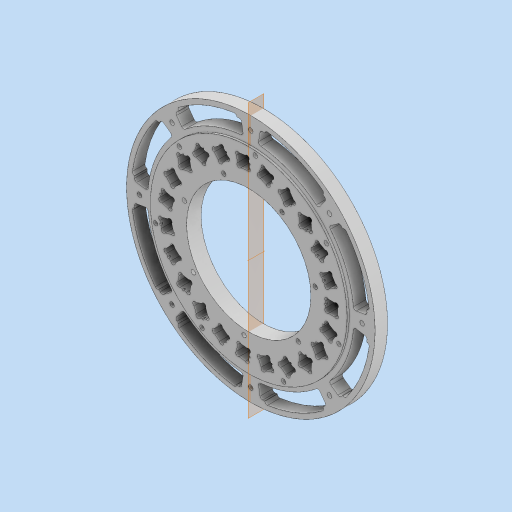
# Autodesk Inventor part: Ring_1050
Saved by Autodesk Inventor 2024.2 (Build 282272000, 272)
## iProperties
Created: 2025-04-23
Part Number: Ring_1050
Material: Generic
Document SubType Name: Modeling
Designer: 23661194
Density: 1 g/cm^3
Appearance: Default
Author: 23661194
Autodesk Inventor part; units mm, degrees
ref_plane "XZ Plane" through (0, 0, 0) normal (0, 1, 0) x (-1, 0, 0)
ref_plane "XY Plane" through (0, 0, 0) normal (0, 0, 1) x (1, 0, 0)
sketch "Shim Tray Slot_1" plane through (0, 0, 0) normal (0, 0, 1) x (1, 0, 0)
  line L0 (30.092, 109.0254) -> (29.9458, 108.3375)
  line L1 (33.5758, 105.3229) -> (31.6829, 97.1237)
  line L2 (-33.5758, 105.3229) -> (-31.6821, 97.1202)
  line L3 (-30.092, 109.0254) -> (-29.9458, 108.3375)
  arc A0 (-32.2001, 107.689) -> (-33.5758, 105.3229) centre (-31.6271, 105.7728) ccw
  arc A1 (29.147, 95.658) -> (-29.1504, 95.657) centre (0, 0) ccw
  arc A2 (28.6337, 111.3782) -> (-28.6337, 111.3782) centre (0, 0) ccw
  arc A3 (-29.9458, 108.3375) -> (-32.2001, 107.689) centre (0, 0) ccw
  arc A4 (32.2001, 107.689) -> (29.9458, 108.3375) centre (0, 0) ccw
  arc A5 (-28.6337, 111.3782) -> (-30.092, 109.0254) centre (-28.1357, 109.4412) ccw
  arc A6 (-31.6821, 97.1202) -> (-29.1504, 95.657) centre (-29.7334, 97.5701) ccw
  arc A7 (29.147, 95.658) -> (31.6829, 97.1237) centre (29.7309, 97.5743) ccw
  arc A8 (33.5758, 105.3229) -> (32.2001, 107.689) centre (31.6271, 105.7728) ccw
  arc A9 (30.092, 109.0254) -> (28.6337, 111.3782) centre (28.1357, 109.4412) ccw
  line L4 (0, 0) -> (0, 107.5)
  arc A10 (33.9656, 105.2329) -> (32.3146, 108.0722) centre (31.6271, 105.7728) ccw
  line L5 (33.9656, 105.2329) -> (32.0726, 97.0337)
  arc A11 (29.0304, 95.2754) -> (32.0726, 97.0337) centre (29.7309, 97.5743) ccw
  arc A12 (29.0304, 95.2754) -> (-29.0338, 95.2743) centre (0, 0) ccw
  arc A13 (-32.0718, 97.0302) -> (-29.0338, 95.2743) centre (-29.7334, 97.5701) ccw
  line L6 (-32.0718, 97.0302) -> (-33.9656, 105.2329)
  arc A14 (-32.3146, 108.0722) -> (-33.9656, 105.2329) centre (-31.6271, 105.7728) ccw
  arc A15 (-30.4152, 108.6221) -> (-32.3146, 108.0722) centre (0, 0) ccw
  line L7 (-30.4152, 108.6221) -> (-30.4833, 108.9422)
  arc A16 (-28.7333, 111.7656) -> (-30.4833, 108.9422) centre (-28.1357, 109.4412) ccw
  arc A17 (28.7333, 111.7656) -> (-28.7333, 111.7656) centre (0, 0) ccw
  arc A18 (30.4833, 108.9422) -> (28.7333, 111.7656) centre (28.1357, 109.4412) ccw
  line L8 (30.4833, 108.9422) -> (30.4152, 108.6221)
  arc A19 (32.3146, 108.0722) -> (30.4152, 108.6221) centre (0, 0) ccw
  dimension "d150" = 22.5
  dimension "d159" = 0.4
  measures "d159" radial gap between concentric circles of A2 A17
sketch "Sketch1" plane through (0, 0, 0) normal (0, 0, 1) x (1, 0, 0)
  circle A0 centre (0, 0) radius 60
  circle A1 centre (0, 0) radius 120
  circle A2 centre (0, 0) radius 95
  dimension "d0" = 120
  dimension "d1" = 240
  dimension "d2" = 190
  constraints: 5 coincident, 3 centre point
  measures "d0" diameter of A0
  measures "d1" diameter of A1
  measures "d2" diameter of A2
extrude "Extrusion1" add sketch "Sketch1" along normal blind 12 contours A1 | A2
extrude "Extrusion2" add sketch "Sketch1" along normal blind 14 contours A2
sketch "Sketch2" plane through (0, 0, 14) normal (0, 0, 1) x (1, 0, 0)
  circle A0 centre (0, 0) radius 80.0067
  circle A1 centre (0, 0) radius 60 projected
  line L0 (80.0067, 0) -> (0, 0)
  line L1 (77.0399, 21.5856) -> (0, 0)
  line L2 (68.3593, 41.5702) -> (0, 0)
  line L3 (54.6089, 58.4718) -> (0, 0)
  line L4 (36.8083, 71.0368) -> (0, 0)
  line L5 (16.2779, 78.3333) -> (0, 0)
  line L6 (-5.4599, 79.8202) -> (0, 0)
  line L7 (-26.7926, 75.3872) -> (0, 0)
  line L8 (-46.1383, 65.3631) -> (0, 0)
  line L9 (-62.0621, 50.4913) -> (0, 0)
  line L10 (-73.3831, 31.8748) -> (0, 0)
  line L11 (-79.2616, 10.8942) -> (0, 0)
  line L12 (-79.2616, -10.8942) -> (0, 0)
  line L13 (-73.3831, -31.8748) -> (0, 0)
  line L14 (-62.0621, -50.4913) -> (0, 0)
  line L15 (-46.1383, -65.3631) -> (0, 0)
  line L16 (-26.7926, -75.3872) -> (0, 0)
  line L17 (-5.4599, -79.8202) -> (0, 0)
  line L18 (16.2779, -78.3333) -> (0, 0)
  line L19 (36.8083, -71.0368) -> (0, 0)
  line L20 (54.6089, -58.4718) -> (0, 0)
  line L21 (68.3593, -41.5702) -> (0, 0)
  line L22 (77.0399, -21.5856) -> (0, 0)
  line L23 (-168, 0) -> (168, 0) projected
  line L24 (85.9467, 5.94) -> (74.0667, 5.94)
  line L25 (74.0667, 5.94) -> (74.0667, -5.94)
  line L26 (74.0667, -5.94) -> (85.9467, -5.94)
  line L27 (85.9467, -5.94) -> (85.9467, 5.94)
  line L28 (85.9467, 5.94) -> (74.0667, -5.94) construction
  line L29 (74.0667, 5.94) -> (85.9467, -5.94) construction
  circle A2 centre (80.0067, 0) radius 2
  circle A3 centre (75.4797, -4.527) radius 2.1
  circle A4 centre (84.5337, -4.527) radius 2.1
  circle A5 centre (84.5337, 4.527) radius 2.1
  circle A6 centre (75.4797, 4.527) radius 2.1
  circle A7 centre (73.7067, 0) radius 0.75
  line L30 (73.7067, 0) -> (80.0067, 0)
  line L31 (79.0288, 29.7471) -> (68.8783, 23.5745)
  line L32 (68.8783, 23.5745) -> (75.0509, 13.424)
  line L33 (75.0509, 13.424) -> (85.2015, 19.5966)
  line L34 (85.2015, 19.5966) -> (79.0288, 29.7471)
  line L35 (79.0288, 29.7471) -> (75.0509, 13.424) construction
  line L36 (68.8783, 23.5745) -> (85.2015, 19.5966) construction
  circle A8 centre (77.0399, 21.5856) radius 2
  circle A9 centre (75.5241, 15.3654) radius 2.1
  circle A10 centre (83.26, 20.0698) radius 2.1
  circle A11 centre (78.5557, 27.8057) radius 2.1
  circle A12 centre (70.8198, 23.1014) radius 2.1
  circle A13 centre (71.657, 18.3122) radius 0.75
  line L37 (71.657, 18.3122) -> (77.0399, 21.5856)
  line L38 (65.8181, 49.577) -> (60.3525, 39.029)
  line L39 (60.3525, 39.029) -> (70.9006, 33.5634)
  line L40 (70.9006, 33.5634) -> (76.3661, 44.1115)
  line L41 (76.3661, 44.1115) -> (65.8181, 49.577)
  line L42 (65.8181, 49.577) -> (70.9006, 33.5634) construction
  line L43 (60.3525, 39.029) -> (76.3661, 44.1115) construction
  circle A14 centre (68.3593, 41.5702) radius 2
  circle A15 centre (70.2961, 35.468) radius 2.1
  circle A16 centre (74.4615, 43.507) radius 2.1
  circle A17 centre (66.4226, 47.6724) radius 2.1
  circle A18 centre (62.2571, 39.6335) radius 2.1
  circle A19 centre (65.4609, 35.9765) radius 0.75
  line L44 (65.4609, 35.9765) -> (68.3593, 41.5702)
  line L45 (48.2773, 63.9926) -> (49.0881, 52.1403)
  line L46 (49.0881, 52.1403) -> (60.9404, 52.951)
  line L47 (60.9404, 52.951) -> (60.1296, 64.8033)
  line L48 (60.1296, 64.8033) -> (48.2773, 63.9926)
  line L49 (48.2773, 63.9926) -> (60.9404, 52.951) construction
  line L50 (49.0881, 52.1403) -> (60.1296, 64.8033) construction
  circle A20 centre (54.6089, 58.4718) radius 2
  circle A21 centre (59.4342, 54.2643) radius 2.1
  circle A22 centre (58.8164, 63.2972) radius 2.1
  circle A23 centre (49.7835, 62.6793) radius 2.1
  circle A24 centre (50.4013, 53.6464) radius 2.1
  circle A25 centre (55.0388, 52.1865) radius 0.75
  line L51 (55.0388, 52.1865) -> (54.6089, 58.4718)
  line L52 (28.53, 72.4641) -> (35.381, 62.7585)
  line L53 (35.381, 62.7585) -> (45.0866, 69.6095)
  line L54 (45.0866, 69.6095) -> (38.2356, 79.3151)
  line L55 (38.2356, 79.3151) -> (28.53, 72.4641)
  line L56 (28.53, 72.4641) -> (45.0866, 69.6095) construction
  line L57 (35.381, 62.7585) -> (38.2356, 79.3151) construction
  circle A26 centre (36.8083, 71.0368) radius 2
  circle A27 centre (43.1174, 69.949) radius 2.1
  circle A28 centre (37.8961, 77.3459) radius 2.1
  circle A29 centre (30.4992, 72.1246) radius 2.1
  circle A30 centre (35.7205, 64.7277) radius 2.1
  circle A31 centre (40.4414, 65.8899) radius 0.75
  line L58 (40.4414, 65.8899) -> (36.8083, 71.0368)
  line L59 (8.4631, 75.2516) -> (19.3596, 70.5186)
  line L60 (19.3596, 70.5186) -> (24.0926, 81.4151)
  line L61 (24.0926, 81.4151) -> (13.1961, 86.1481)
  line L62 (13.1961, 86.1481) -> (8.4631, 75.2516)
  line L63 (8.4631, 75.2516) -> (24.0926, 81.4151) construction
  line L64 (19.3596, 70.5186) -> (13.1961, 86.1481) construction
  circle A32 centre (16.2779, 78.3333) radius 2
  circle A33 centre (22.2336, 80.682) radius 2.1
  circle A34 centre (13.9292, 84.2891) radius 2.1
  circle A35 centre (10.3221, 75.9847) radius 2.1
  circle A36 centre (18.6265, 72.3775) radius 2.1
  circle A37 centre (22.0563, 75.8234) radius 0.75
  line L65 (22.0563, 75.8234) -> (16.2779, 78.3333)
  line L66 (-10.5357, 73.1267) -> (1.2337, 74.7444)
  line L67 (1.2337, 74.7444) -> (-0.384, 86.5137)
  line L68 (-0.384, 86.5137) -> (-12.1534, 84.8961)
  line L69 (-12.1534, 84.8961) -> (-10.5357, 73.1267)
  line L70 (-10.5357, 73.1267) -> (-0.384, 86.5137) construction
  line L71 (1.2337, 74.7444) -> (-12.1534, 84.8961) construction
  circle A38 centre (-5.4599, 79.8202) radius 2
  circle A39 centre (-1.5914, 84.9215) radius 2.1
  circle A40 centre (-10.5611, 83.6886) radius 2.1
  circle A41 centre (-9.3283, 74.719) radius 2.1
  circle A42 centre (-0.3586, 75.9518) radius 2.1
  circle A43 centre (0.7815, 80.6781) radius 0.75
  line L72 (0.7815, 80.6781) -> (-5.4599, 79.8202)
  line L73 (-27.6517, 67.0308) -> (-18.4362, 74.5282)
  line L74 (-18.4362, 74.5282) -> (-25.9336, 83.7436)
  line L75 (-25.9336, 83.7436) -> (-35.149, 76.2463)
  line L76 (-35.149, 76.2463) -> (-27.6517, 67.0308)
  line L77 (-27.6517, 67.0308) -> (-25.9336, 83.7436) construction
  line L78 (-18.4362, 74.5282) -> (-35.149, 76.2463) construction
  circle A44 centre (-26.7926, 75.3872) radius 2
  circle A45 centre (-26.1379, 81.7558) radius 2.1
  circle A46 centre (-33.1612, 76.0419) radius 2.1
  circle A47 centre (-27.4473, 69.0186) radius 2.1
  circle A48 centre (-20.424, 74.7325) radius 2.1
  circle A49 centre (-21.9056, 79.3631) radius 0.75
  line L79 (-21.9056, 79.3631) -> (-26.7926, 75.3872)
  line L80 (-42.5305, 57.7769) -> (-38.5521, 68.9709)
  line L81 (-38.5521, 68.9709) -> (-49.7462, 72.9493)
  line L82 (-49.7462, 72.9493) -> (-53.7245, 61.7553)
  line L83 (-53.7245, 61.7553) -> (-42.5305, 57.7769)
  line L84 (-42.5305, 57.7769) -> (-49.7462, 72.9493) construction
  line L85 (-38.5521, 68.9709) -> (-53.7245, 61.7553) construction
  circle A50 centre (-46.1383, 65.3631) radius 2
  circle A51 centre (-48.8879, 71.1447) radius 2.1
  circle A52 centre (-51.9199, 62.6135) radius 2.1
  circle A53 centre (-43.3887, 59.5815) radius 2.1
  circle A54 centre (-40.3567, 68.1127) radius 2.1
  circle A55 centre (-44.0286, 71.2993) radius 0.75
  line L86 (-44.0286, 71.2993) -> (-46.1383, 65.3631)
  line L87 (-55.0378, 45.8841) -> (-57.4549, 57.5156)
  line L88 (-57.4549, 57.5156) -> (-69.0864, 55.0985)
  line L89 (-69.0864, 55.0985) -> (-66.6694, 43.467)
  line L90 (-66.6694, 43.467) -> (-55.0378, 45.8841)
  line L91 (-55.0378, 45.8841) -> (-69.0864, 55.0985) construction
  line L92 (-57.4549, 57.5156) -> (-66.6694, 43.467) construction
  circle A56 centre (-62.0621, 50.4913) radius 2
  circle A57 centre (-67.4155, 54.0026) radius 2.1
  circle A58 centre (-65.5734, 45.1379) radius 2.1
  circle A59 centre (-56.7088, 46.98) radius 2.1
  circle A60 centre (-58.5509, 55.8446) radius 2.1
  circle A61 centre (-63.3439, 56.6595) radius 0.75
  line L93 (-63.3439, 56.6595) -> (-62.0621, 50.4913)
  line L94 (-64.9876, 31.588) -> (-73.0963, 40.2703)
  line L95 (-73.0963, 40.2703) -> (-81.7786, 32.1616)
  line L96 (-81.7786, 32.1616) -> (-73.6699, 23.4792)
  line L97 (-73.6699, 23.4792) -> (-64.9876, 31.588)
  line L98 (-64.9876, 31.588) -> (-81.7786, 32.1616) construction
  line L99 (-73.0963, 40.2703) -> (-73.6699, 23.4792) construction
  circle A62 centre (-73.3831, 31.8748) radius 2
  circle A63 centre (-79.7815, 32.0933) radius 2.1
  circle A64 centre (-73.6017, 25.4764) radius 2.1
  circle A65 centre (-66.9847, 31.6562) radius 2.1
  circle A66 centre (-73.1645, 38.2732) radius 2.1
  circle A67 centre (-77.6832, 36.479) radius 0.75
  line L100 (-77.6832, 36.479) -> (-73.3831, 31.8748)
  line L101 (-71.9392, 15.0114) -> (-83.3787, 18.2166)
  line L102 (-83.3787, 18.2166) -> (-86.5839, 6.7771)
  line L103 (-86.5839, 6.7771) -> (-75.1444, 3.5719)
  line L104 (-75.1444, 3.5719) -> (-71.9392, 15.0114)
  line L105 (-71.9392, 15.0114) -> (-86.5839, 6.7771) construction
  line L106 (-83.3787, 18.2166) -> (-75.1444, 3.5719) construction
  circle A68 centre (-79.2616, 10.8942) radius 2
  circle A69 centre (-84.842, 7.7565) radius 2.1
  circle A70 centre (-76.1238, 5.3138) radius 2.1
  circle A71 centre (-73.6811, 14.032) radius 2.1
  circle A72 centre (-82.3993, 16.4747) radius 2.1
  circle A73 centre (-85.3279, 12.594) radius 0.75
  line L107 (-85.3279, 12.594) -> (-79.2616, 10.8942)
  line L108 (-75.1444, -3.5719) -> (-86.5839, -6.7771)
  line L109 (-86.5839, -6.7771) -> (-83.3787, -18.2166)
  line L110 (-83.3787, -18.2166) -> (-71.9392, -15.0114)
  line L111 (-71.9392, -15.0114) -> (-75.1444, -3.5719)
  line L112 (-75.1444, -3.5719) -> (-83.3787, -18.2166) construction
  line L113 (-86.5839, -6.7771) -> (-71.9392, -15.0114) construction
  circle A74 centre (-79.2616, -10.8942) radius 2
  circle A75 centre (-82.3993, -16.4747) radius 2.1
  circle A76 centre (-73.6811, -14.032) radius 2.1
  circle A77 centre (-76.1238, -5.3138) radius 2.1
  circle A78 centre (-84.842, -7.7565) radius 2.1
  circle A79 centre (-85.3279, -12.594) radius 0.75
  line L114 (-85.3279, -12.594) -> (-79.2616, -10.8942)
  line L115 (-73.6699, -23.4792) -> (-81.7786, -32.1616)
  line L116 (-81.7786, -32.1616) -> (-73.0963, -40.2703)
  line L117 (-73.0963, -40.2703) -> (-64.9876, -31.588)
  line L118 (-64.9876, -31.588) -> (-73.6699, -23.4792)
  line L119 (-73.6699, -23.4792) -> (-73.0963, -40.2703) construction
  line L120 (-81.7786, -32.1616) -> (-64.9876, -31.588) construction
  circle A80 centre (-73.3831, -31.8748) radius 2
  circle A81 centre (-73.1645, -38.2732) radius 2.1
  circle A82 centre (-66.9847, -31.6562) radius 2.1
  circle A83 centre (-73.6017, -25.4764) radius 2.1
  circle A84 centre (-79.7815, -32.0934) radius 2.1
  circle A85 centre (-77.6832, -36.479) radius 0.75
  line L121 (-77.6832, -36.479) -> (-73.3831, -31.8748)
  line L122 (-66.6694, -43.467) -> (-69.0864, -55.0985)
  line L123 (-69.0864, -55.0985) -> (-57.4549, -57.5156)
  line L124 (-57.4549, -57.5156) -> (-55.0378, -45.8841)
  line L125 (-55.0378, -45.8841) -> (-66.6694, -43.467)
  line L126 (-66.6694, -43.467) -> (-57.4549, -57.5156) construction
  line L127 (-69.0864, -55.0985) -> (-55.0378, -45.8841) construction
  circle A86 centre (-62.0621, -50.4913) radius 2
  circle A87 centre (-58.5509, -55.8446) radius 2.1
  circle A88 centre (-56.7088, -46.98) radius 2.1
  circle A89 centre (-65.5734, -45.1379) radius 2.1
  circle A90 centre (-67.4155, -54.0026) radius 2.1
  circle A91 centre (-63.3439, -56.6595) radius 0.75
  line L128 (-63.3439, -56.6595) -> (-62.0621, -50.4913)
  line L129 (-53.7245, -61.7553) -> (-49.7462, -72.9493)
  line L130 (-49.7462, -72.9493) -> (-38.5521, -68.9709)
  line L131 (-38.5521, -68.9709) -> (-42.5305, -57.7769)
  line L132 (-42.5305, -57.7769) -> (-53.7245, -61.7553)
  line L133 (-53.7245, -61.7553) -> (-38.5521, -68.9709) construction
  line L134 (-49.7462, -72.9493) -> (-42.5305, -57.7769) construction
  circle A92 centre (-46.1383, -65.3631) radius 2
  circle A93 centre (-40.3567, -68.1127) radius 2.1
  circle A94 centre (-43.3887, -59.5815) radius 2.1
  circle A95 centre (-51.9199, -62.6135) radius 2.1
  circle A96 centre (-48.8879, -71.1447) radius 2.1
  circle A97 centre (-44.0286, -71.2993) radius 0.75
  line L135 (-44.0286, -71.2993) -> (-46.1383, -65.3631)
  line L136 (-35.149, -76.2463) -> (-25.9336, -83.7436)
  line L137 (-25.9336, -83.7436) -> (-18.4362, -74.5282)
  line L138 (-18.4362, -74.5282) -> (-27.6517, -67.0308)
  line L139 (-27.6517, -67.0308) -> (-35.149, -76.2463)
  line L140 (-35.149, -76.2463) -> (-18.4362, -74.5282) construction
  line L141 (-25.9336, -83.7436) -> (-27.6517, -67.0308) construction
  circle A98 centre (-26.7926, -75.3872) radius 2
  circle A99 centre (-20.424, -74.7325) radius 2.1
  circle A100 centre (-27.4473, -69.0186) radius 2.1
  circle A101 centre (-33.1612, -76.0419) radius 2.1
  circle A102 centre (-26.1379, -81.7558) radius 2.1
  circle A103 centre (-21.9056, -79.3631) radius 0.75
  line L142 (-21.9056, -79.3631) -> (-26.7926, -75.3872)
  line L143 (-12.1534, -84.8961) -> (-0.384, -86.5137)
  line L144 (-0.384, -86.5137) -> (1.2337, -74.7444)
  line L145 (1.2337, -74.7444) -> (-10.5357, -73.1267)
  line L146 (-10.5357, -73.1267) -> (-12.1534, -84.8961)
  line L147 (-12.1534, -84.8961) -> (1.2337, -74.7444) construction
  line L148 (-0.384, -86.5137) -> (-10.5357, -73.1267) construction
  circle A104 centre (-5.4599, -79.8202) radius 2
  circle A105 centre (-0.3586, -75.9518) radius 2.1
  circle A106 centre (-9.3283, -74.719) radius 2.1
  circle A107 centre (-10.5611, -83.6886) radius 2.1
  circle A108 centre (-1.5914, -84.9215) radius 2.1
  circle A109 centre (0.7815, -80.6781) radius 0.75
  line L149 (0.7815, -80.6781) -> (-5.4599, -79.8202)
  line L150 (13.1961, -86.1481) -> (24.0926, -81.4151)
  line L151 (24.0926, -81.4151) -> (19.3596, -70.5186)
  line L152 (19.3596, -70.5186) -> (8.4631, -75.2516)
  line L153 (8.4631, -75.2516) -> (13.1961, -86.1481)
  line L154 (13.1961, -86.1481) -> (19.3596, -70.5186) construction
  line L155 (24.0926, -81.4151) -> (8.4631, -75.2516) construction
  circle A110 centre (16.2779, -78.3333) radius 2
  circle A111 centre (18.6265, -72.3775) radius 2.1
  circle A112 centre (10.3221, -75.9847) radius 2.1
  circle A113 centre (13.9292, -84.2891) radius 2.1
  circle A114 centre (22.2336, -80.682) radius 2.1
  circle A115 centre (22.0563, -75.8234) radius 0.75
  line L156 (22.0563, -75.8234) -> (16.2779, -78.3333)
  line L157 (38.2356, -79.3151) -> (45.0866, -69.6095)
  line L158 (45.0866, -69.6095) -> (35.381, -62.7585)
  line L159 (35.381, -62.7585) -> (28.53, -72.4641)
  line L160 (28.53, -72.4641) -> (38.2356, -79.3151)
  line L161 (38.2356, -79.3151) -> (35.381, -62.7585) construction
  line L162 (45.0866, -69.6095) -> (28.53, -72.4641) construction
  circle A116 centre (36.8083, -71.0368) radius 2
  circle A117 centre (35.7205, -64.7277) radius 2.1
  circle A118 centre (30.4992, -72.1246) radius 2.1
  circle A119 centre (37.8961, -77.3459) radius 2.1
  circle A120 centre (43.1174, -69.949) radius 2.1
  circle A121 centre (40.4414, -65.8899) radius 0.75
  line L163 (40.4414, -65.8899) -> (36.8083, -71.0368)
  line L164 (60.1296, -64.8033) -> (60.9404, -52.951)
  line L165 (60.9404, -52.951) -> (49.0881, -52.1403)
  line L166 (49.0881, -52.1403) -> (48.2773, -63.9926)
  line L167 (48.2773, -63.9926) -> (60.1296, -64.8033)
  line L168 (60.1296, -64.8033) -> (49.0881, -52.1403) construction
  line L169 (60.9404, -52.951) -> (48.2773, -63.9926) construction
  circle A122 centre (54.6089, -58.4718) radius 2
  circle A123 centre (50.4013, -53.6464) radius 2.1
  circle A124 centre (49.7835, -62.6793) radius 2.1
  circle A125 centre (58.8164, -63.2972) radius 2.1
  circle A126 centre (59.4342, -54.2643) radius 2.1
  circle A127 centre (55.0388, -52.1865) radius 0.75
  line L170 (55.0388, -52.1865) -> (54.6089, -58.4718)
  line L171 (76.3661, -44.1115) -> (70.9006, -33.5634)
  line L172 (70.9006, -33.5634) -> (60.3525, -39.029)
  line L173 (60.3525, -39.029) -> (65.8181, -49.577)
  line L174 (65.8181, -49.577) -> (76.3661, -44.1115)
  line L175 (76.3661, -44.1115) -> (60.3525, -39.029) construction
  line L176 (70.9006, -33.5634) -> (65.8181, -49.577) construction
  circle A128 centre (68.3593, -41.5702) radius 2
  circle A129 centre (62.2571, -39.6335) radius 2.1
  circle A130 centre (66.4226, -47.6724) radius 2.1
  circle A131 centre (74.4615, -43.507) radius 2.1
  circle A132 centre (70.2961, -35.468) radius 2.1
  circle A133 centre (65.4609, -35.9765) radius 0.75
  line L177 (65.4609, -35.9765) -> (68.3593, -41.5702)
  line L178 (85.2015, -19.5966) -> (75.0509, -13.424)
  line L179 (75.0509, -13.424) -> (68.8783, -23.5745)
  line L180 (68.8783, -23.5745) -> (79.0288, -29.7471)
  line L181 (79.0288, -29.7471) -> (85.2015, -19.5966)
  line L182 (85.2015, -19.5966) -> (68.8783, -23.5745) construction
  line L183 (75.0509, -13.424) -> (79.0288, -29.7471) construction
  circle A134 centre (77.0399, -21.5856) radius 2
  circle A135 centre (70.8198, -23.1014) radius 2.1
  circle A136 centre (78.5557, -27.8057) radius 2.1
  circle A137 centre (83.26, -20.0698) radius 2.1
  circle A138 centre (75.5241, -15.3654) radius 2.1
  circle A139 centre (71.657, -18.3122) radius 0.75
  line L184 (71.657, -18.3122) -> (77.0399, -21.5856)
  point P0 (76.4941, -28.2058)
  point P1 (80.5702, -27.2125)
  point P2 (83.6601, -22.1313)
  point P3 (82.6668, -18.0553)
  point P4 (77.5856, -14.9653)
  point P5 (73.5096, -15.9586)
  point P6 (70.4196, -21.0398)
  point P7 (71.4129, -25.1158)
  point P8 (61.7173, -41.6629)
  point P9 (64.4533, -46.9431)
  point P10 (68.452, -48.2122)
  point P11 (73.7322, -45.4763)
  point P12 (75.0013, -41.4775)
  point P13 (72.2654, -36.1973)
  point P14 (68.2666, -34.9282)
  point P15 (62.9864, -37.6642)
  point P16 (60.7379, -55.9106)
  point P17 (57.9808, -52.7486)
  point P18 (52.0477, -52.3427)
  point P19 (48.8856, -55.0999)
  point P20 (48.4798, -61.033)
  point P21 (51.2369, -64.195)
  point P22 (57.17, -64.6009)
  point P23 (60.3321, -61.8437)
  point P24 (30.2408, -70.0406)
  point P25 (30.9536, -74.1749)
  point P26 (35.8121, -77.6043)
  point P27 (39.9464, -76.8915)
  point P28 (43.3759, -72.033)
  point P29 (42.663, -67.8987)
  point P30 (37.8045, -64.4693)
  point P31 (33.6702, -65.1821)
  point P32 (12.0143, -83.4271)
  point P33 (15.917, -84.9662)
  point P34 (21.3717, -82.5969)
  point P35 (22.9107, -78.6941)
  point P36 (20.5415, -73.2395)
  point P37 (16.6387, -71.7005)
  point P38 (11.184, -74.0697)
  point P39 (9.645, -77.9725)
  point P40 (0.8297, -77.6833)
  point P41 (-1.7052, -74.3404)
  point P42 (-7.5968, -73.5307)
  point P43 (-10.9396, -76.0656)
  point P44 (-11.7494, -81.9572)
  point P45 (-9.2145, -85.3)
  point P46 (-3.3229, -86.1098)
  point P47 (0.0199, -83.5748)
  point P48 (-25.3505, -68.903)
  point P49 (-29.5238, -69.332)
  point P50 (-33.2769, -73.9451)
  point P51 (-32.8478, -78.1184)
  point P52 (-28.2347, -81.8715)
  point P53 (-24.0614, -81.4424)
  point P54 (-20.3084, -76.8293)
  point P55 (-20.7374, -72.656)
  point P56 (-52.7311, -64.5505)
  point P57 (-50.7396, -70.1541)
  point P58 (-46.9509, -71.9559)
  point P59 (-41.3473, -69.9644)
  point P60 (-39.5455, -66.1757)
  point P61 (-41.537, -60.5721)
  point P62 (-45.3257, -58.7703)
  point P63 (-50.9293, -60.7618)
  point P64 (-56.8513, -54.6111)
  point P65 (-55.6414, -48.7885)
  point P66 (-57.9423, -45.2805)
  point P67 (-63.7649, -44.0706)
  point P68 (-67.2729, -46.3715)
  point P69 (-68.4829, -52.194)
  point P70 (-66.1819, -55.7021)
  point P71 (-60.3594, -56.912)
  point P72 (-71.5019, -25.504)
  point P73 (-75.6947, -25.6473)
  point P74 (-79.7538, -29.9935)
  point P75 (-79.6106, -34.1864)
  point P76 (-75.2643, -38.2455)
  point P77 (-71.0715, -38.1023)
  point P78 (-67.0124, -33.756)
  point P79 (-67.1556, -29.5631)
  point P80 (-74.3441, -6.4284)
  point P81 (-78.0009, -4.3723)
  point P82 (-83.7274, -5.9768)
  point P83 (-85.7835, -9.6336)
  point P84 (-84.179, -15.3601)
  point P85 (-80.5222, -17.4162)
  point P86 (-74.7957, -15.8117)
  point P87 (-72.7396, -12.1549)
  point P88 (-72.7396, 12.1549)
  point P89 (-74.7957, 15.8117)
  point P90 (-80.5222, 17.4162)
  point P91 (-84.179, 15.3601)
  point P92 (-85.7835, 9.6336)
  point P93 (-83.7274, 5.9768)
  point P94 (-78.0009, 4.3723)
  point P95 (-74.3441, 6.4284)
  point P96 (-67.1556, 29.5632)
  point P97 (-67.0124, 33.756)
  point P98 (-71.0715, 38.1023)
  point P99 (-75.2643, 38.2455)
  point P100 (-79.6106, 34.1864)
  point P101 (-79.7538, 29.9935)
  point P102 (-75.6947, 25.6473)
  point P103 (-71.5018, 25.504)
  point P104 (-57.9423, 45.2805)
  point P105 (-55.6414, 48.7885)
  point P106 (-56.8513, 54.6111)
  point P107 (-60.3594, 56.912)
  point P108 (-66.1819, 55.7021)
  point P109 (-68.4829, 52.194)
  point P110 (-67.2729, 46.3715)
  point P111 (-63.7649, 44.0706)
  point P112 (-45.3257, 58.7703)
  point P113 (-41.537, 60.5721)
  point P114 (-39.5455, 66.1757)
  point P115 (-41.3473, 69.9644)
  point P116 (-46.9509, 71.9559)
  point P117 (-50.7396, 70.1541)
  point P118 (-52.7311, 64.5505)
  point P119 (-50.9293, 60.7618)
  point P120 (-20.7374, 72.656)
  point P121 (-20.3084, 76.8293)
  point P122 (-24.0614, 81.4424)
  point P123 (-28.2347, 81.8715)
  point P124 (-32.8478, 78.1184)
  point P125 (-33.2769, 73.9451)
  point P126 (-29.5238, 69.332)
  point P127 (-25.3505, 68.903)
  point P128 (-10.9396, 76.0656)
  point P129 (-7.5968, 73.5307)
  point P130 (-1.7052, 74.3404)
  point P131 (0.8297, 77.6833)
  point P132 (0.0199, 83.5748)
  point P133 (-3.3229, 86.1098)
  point P134 (-9.2145, 85.3)
  point P135 (-11.7494, 81.9572)
  point P136 (9.645, 77.9725)
  point P137 (11.184, 74.0697)
  point P138 (16.6387, 71.7005)
  point P139 (20.5415, 73.2395)
  point P140 (22.9107, 78.6941)
  point P141 (21.3717, 82.5969)
  point P142 (15.917, 84.9662)
  point P143 (12.0143, 83.4271)
  point P144 (30.2408, 70.0406)
  point P145 (33.6702, 65.1821)
  point P146 (37.8045, 64.4693)
  point P147 (42.663, 67.8987)
  point P148 (43.3759, 72.033)
  point P149 (39.9464, 76.8915)
  point P150 (35.8121, 77.6043)
  point P151 (30.9536, 74.1749)
  point P152 (60.7379, 55.9106)
  point P153 (60.3321, 61.8437)
  point P154 (57.17, 64.6009)
  point P155 (51.2369, 64.195)
  point P156 (48.4798, 61.033)
  point P157 (48.8856, 55.0999)
  point P158 (52.0477, 52.3427)
  point P159 (57.9808, 52.7486)
  point P160 (72.2654, 36.1973)
  point P161 (75.0013, 41.4775)
  point P162 (73.7322, 45.4763)
  point P163 (68.452, 48.2122)
  point P164 (64.4533, 46.9431)
  point P165 (61.7173, 41.6629)
  point P166 (62.9864, 37.6642)
  point P167 (68.2666, 34.9282)
  point P168 (71.4129, 25.1158)
  point P169 (70.4196, 21.0398)
  point P170 (73.5096, 15.9586)
  point P171 (77.5856, 14.9653)
  point P172 (82.6668, 18.0553)
  point P173 (83.6601, 22.1313)
  point P174 (80.5702, 27.2125)
  point P175 (76.4941, 28.2058)
  point P176 (77.0333, 5.94)
  point P177 (74.0667, 2.9735)
  point P178 (74.0667, -2.9735)
  point P179 (77.0333, -5.94)
  point P180 (82.9802, -5.94)
  point P181 (85.9467, -2.9735)
  point P182 (85.9467, 2.9735)
  point P183 (82.9802, 5.94)
  dimension "d7" = 160.0135
  dimension "d93" = -31.304
  dimension "d94" = -62.609
  dimension "d95" = -93.913
  dimension "d96" = -125.217
  dimension "d97" = -156.522
  dimension "d98" = -187.826
  dimension "d99" = -219.13
  dimension "d100" = -250.435
  dimension "d101" = -281.739
  dimension "d103" = -344.348
  dimension "d104" = -15.652
  dimension "d105" = -46.957
  dimension "d106" = -78.261
  dimension "d107" = -109.565
  dimension "d108" = -140.87
  dimension "d109" = -172.174
  dimension "d110" = -203.478
  dimension "d111" = -234.783
  dimension "d112" = -266.087
  dimension "d113" = -297.391
  dimension "d114" = -328.696
  dimension "d10" = 360
  dimension "d92" = 0
  dimension "d102" = -313.043
  constraints: 46 end point, 1 coincident, 1 horizontal, 1 horizontal alignment, 96 other
  measures "d92" vertical extent of L0
extrude "Extrusion3" cut sketch "Sketch2" against normal blind 12 contours L0 A2 A0 | L23 A2 A0 | A0 A2 L0 | A0 A2 L23 | A2 L0 A7 L25 A6 L24 A0 | A0 L24 A5 L27 L23 A2 | A2 L23 L27 A4 L26 A0 | A0 L26 A3 L25 A7 L0 A2 | A7 L25 L0 | L0 L25 A7 | L33 A9 L32 A13 L37 A8 A0 | A0 A8 L31 A11 L34 A10 L33 | A5 L27 L24 | L24 L27 A5 | A6 L25 L24 | L24 L25 A6 | L178 A137 L181 A136 L180 A0 A134 | A0 A134 L184 A139 L179 A138 L178 | A3 L25 L26 | L26 L25 A3 | A4 L27 L26 | L26 L27 A4 | A8 L37 A0 | A0 A8 | A9 L32 L33 | L33 L32 A9 | A10 L34 L33 | L33 L34 A10 | A134 A0 | A0 L184 A134 | A137 L181 L178 | L178 L181 A137 | A138 L179 L178 | L178 L179 A138 | L1 A8 A0 | L37 A8 L1 | L37 A13 L32 L1 A8 | A0 A134 L22 | L22 A134 L184 | A134 L22 L179 A139 L184 | A8 L1 L32 A12 L31 A0 | L37 L32 A13 | A13 L32 L37 | A11 L31 L34 | L34 L31 A11 | A0 L180 A135 L179 L22 A134 | L184 L179 A139 | A139 L179 L184 | A136 L180 L181 | L181 L180 A136 | A15 L39 L40 A0 | A0 L40 A15 | A12 L32 L31 | L31 L32 A12 | A132 L171 A0 | A0 L171 L172 A132 | A135 L179 L180 | L180 L179 A135 | A18 L38 L39 L2 | L2 L39 A18 | A129 L172 L21 | L21 L172 L173 A129 | A24 L45 L3 | L3 L45 L46 A24 | A30 L52 L4 | L4 L52 L53 A30 | L59 A35 L62 A0 A32 L5 | L5 A32 L65 A37 L60 A36 L59 | L66 A41 L69 A0 A38 L6 | L6 A38 A0 A43 L67 A42 L66 | L73 A47 L76 A0 A44 L7 | L7 A44 A0 L74 A48 L73 | A53 L83 L80 L8 | L8 L80 A53 | A59 L90 L9 | L9 L90 L87 A59 | L97 A64 L96 A0 A62 L10 | L10 A62 A0 L94 A65 L97 | L104 A70 L103 A0 A68 L11 | L11 A68 A0 L101 A71 L104 | L111 A76 L110 A0 A74 L12 | L12 A74 A0 L108 A77 L111 | L118 A82 L117 A0 A80 L13 | L13 A80 A0 L115 A83 L118 | A88 L124 L125 L14 | L14 L125 A88 | A94 L131 L15 | L15 L131 L132 A94 | L138 A99 L137 A0 A98 L16 | L16 A98 A0 L139 A100 L138 | L145 A105 L144 A109 A0 A104 L17 | L17 A104 A0 L146 A106 L145 | L152 A111 L151 A115 L156 A110 L18 | L18 A110 A0 L153 A112 L152 | A117 L158 L159 L19 | L19 L159 A117 | A123 L165 L166 L20 | L20 L166 A123 | L40 L39 A15 A0 | A0 A15 L40 | L39 A19 L44 A14 A0 A15 | L171 A132 A0 | A0 A132 L172 L171 | A132 A0 A128 L177 A133 L172 | L39 L38 A18 L2 | L2 A18 L39 | L38 A17 A0 A14 L2 A18 | A18 L2 A14 L44 A19 L39 | L172 A129 L21 | L21 A129 L173 L172 | L172 A133 L177 A128 L21 A129 | A129 L21 A128 A0 A130 L173 | L45 A24 L3 | L3 A24 L46 L45 | L45 A23 A0 A20 L3 A24 | A24 L3 A20 L51 A25 L46 | L52 A30 L4 | L4 A30 L53 L52 | L52 A29 A0 A26 L4 A30 | A30 L4 A26 L58 A31 L53 | A32 A0 L5 | L5 L65 A32 | A35 L62 L59 | L59 L62 A35 | A36 L60 L59 | L59 L60 A36 | A38 A0 L6 | L6 A0 A38 | A41 L69 L66 | L66 L69 A41 | A42 L67 L66 | L66 L67 A42 | A44 A0 L7 | L7 A0 A44 | A47 L76 L73 | L73 L76 A47 | A48 L74 L73 | L73 L74 A48 | L80 L83 A53 L8 | L8 A53 L80 | L83 A52 A0 A50 L8 A53 | L90 A59 L9 | L9 A59 L87 L90 | L90 A58 A0 A56 L9 A59 | A62 A0 L10 | L10 A0 A62 | A64 L96 L97 | L97 L96 A64 | A65 L94 L97 | L97 L94 A65 | A68 A0 L11 | L11 A0 A68 | A70 L103 L104 | L104 L103 A70 | A71 L101 L104 | L104 L101 A71 | A74 A0 L12 | L12 A0 A74 | A76 L110 L111 | L111 L110 A76 | A77 L108 L111 | L111 L108 A77 | A80 A0 L13 | L13 A0 A80 | A82 L117 L118 | L118 L117 A82 | A83 L115 L118 | L118 L115 A83 | L125 L124 A88 L14 | L14 A88 L125 | A88 L14 A86 A0 A89 L125 | L131 A94 L15 | L15 A94 L132 L131 | A94 L15 A92 A0 A95 L132 | A98 A0 L16 | L16 A0 A98 | A99 L137 L138 | L138 L137 A99 | A100 L139 L138 | L138 L139 A100 | A104 A0 L17 | L17 A0 A104 | A105 L144 L145 | L145 L144 A105 | A106 L146 L145 | L145 L146 A106 | A110 L156 L18 | L18 A0 A110 | A111 L151 L152 | L152 L151 A111 | A112 L153 L152 | L152 L153 A112 | L159 L158 A117 L19 | L19 A117 L159 | L158 A121 L163 A116 L19 A117 | A117 L19 A116 A0 A118 L159 | L166 L165 A123 L20 | L20 A123 L166 | L165 A127 L170 A122 L20 A123 | A123 L20 A122 A0 A124 L166 | L103 A69 L102 A73 L107 A68 A0 | A0 A74 L114 A79 L109 A78 L108 | A0 A14 A17 L41 A16 L40 A15 | L39 L44 A19 | A132 L171 A131 L174 A130 A0 A128 | A133 L177 L172 | A17 A0 L38 | L38 A0 A17 | A19 L44 L39 | L172 L177 A133 | A130 A0 L173 | L173 A0 A130 | A23 A0 L45 | L45 A0 A23 | A25 L51 L46 | A29 A0 L55 L52 | L52 L55 A0 A29 | A31 L58 L53 | A0 A32 | A0 A32 L65 | A0 L62 A34 L61 A33 L60 A32 | A32 A0 L60 A37 L65 | L72 A38 A0 | A0 A38 L72 | A0 L69 A40 L68 A39 L67 A43 L72 A38 | L79 A44 A0 | A0 A44 L79 | A0 L76 A46 L75 A45 L74 A49 L79 A44 | L8 A50 A0 A54 L80 A53 | A52 A0 L83 | L83 A0 A52 | L9 A56 A0 A60 L87 A59 | A58 A0 L89 L90 | L90 L89 A0 A58 | L100 A62 A0 | A0 A62 L100 | A0 L96 A63 L95 A67 L100 A62 | L107 A68 A0 | A0 A68 L107 | L114 A74 A0 | A0 A74 L114 | L121 A80 A0 | A0 A80 L121 | A80 L121 A85 L116 A84 L115 A0 | A88 L124 A87 A0 A86 L14 | A89 A0 L122 L125 | L125 L122 A0 A89 | A94 L131 A93 A0 A92 L15 | A95 A0 L132 | L132 A0 A95 | L142 A98 A0 | A0 A98 L142 | A98 L142 A103 L137 A102 L136 A101 L139 A0 | L149 A104 A0 | A0 A104 L149 | A104 L149 A109 L144 A108 L143 A107 L146 A0 | A0 A110 | L156 A110 A0 | L156 A115 L151 A0 A110 | A110 A0 L151 A114 L150 A113 L153 | L158 L163 A121 | A118 A0 L160 L159 | L159 L160 A0 A118 | L165 L170 A127 | A124 A0 L166 | L166 A0 A124 | A69 L102 L103 | L103 L102 A69 | A78 L109 L108 | L108 L109 A78 | A14 L44 A0 | A0 A14 | A16 L41 L40 | L40 L41 A16 | A128 A0 | A0 L177 A128 | A131 L174 L171 | L171 L174 A131 | A14 A0 L2 | L2 L44 A14 | L38 L41 A17 A0 | A0 A17 L41 L38 | A128 L177 L21 | L21 A0 A128 | L173 L174 A130 A0 | A0 A130 L174 L173 | A20 A0 L3 | L3 L51 A20 | L45 L48 A23 A0 | A0 A23 L48 L45 | A23 L48 A22 L47 A21 A0 A20 | L51 A25 L46 | L51 A20 A0 A21 L46 A25 | A26 A0 L4 | L4 L58 A26 | A29 L55 A0 | L58 A31 L53 | L58 A26 A0 L53 A31 | L65 L60 A37 | A37 L60 L65 | A38 L72 A43 A0 | A43 A0 L67 | A44 L79 A49 L74 A0 | A50 A0 L8 | L8 A0 A50 | A54 A0 L81 L80 | L80 L81 A0 A54 | L83 L82 A52 A0 | A0 A52 L82 L83 | A52 L82 A51 L81 A55 L86 A50 A0 | A56 A0 L9 | L9 A0 A56 | A58 L89 A0 | A60 A0 L87 | L87 A0 A60 | A62 L100 A67 L95 A66 L94 A0 | A68 L107 A73 L102 A72 L101 A0 | A0 L110 A75 L109 A79 L114 A74 | A0 L117 A81 L116 A85 L121 A80 | A86 A0 L14 | L14 A0 A86 | A87 A0 L124 | L124 A0 A87 | A0 L122 A89 | A92 A0 L15 | L15 A0 A92 | A93 A0 L130 L131 | L131 L130 A0 A93 | L132 L129 A95 A0 | A0 A95 L129 L132 | A0 A92 L135 A97 L130 A96 L129 A95 | A0 L137 A103 L142 A98 | A0 A109 L149 A104 | L144 A0 A109 | L156 L151 A115 | A115 L151 L156 | A116 L163 L19 | L19 A0 A116 | L158 A121 L163 | A121 L158 A0 A116 L163 | A0 L160 A118 | A122 L170 L20 | L20 A0 A122 | L165 A127 L170 | A127 L165 A126 A0 A122 L170 | L166 L167 A124 A0 | A0 A124 L167 L166 | A0 A122 A126 L164 A125 L167 A124 | A21 L46 A0 | A0 L46 L47 A21 | A126 L164 L165 A0 | A0 L165 A126 | A0 A20 | A0 A20 L51 | A0 A26 A29 L55 A28 L54 A27 L53 | A0 A26 | A0 A26 L58 | L55 A29 A0 | A34 L61 L62 | L62 L61 A34 | A43 L72 L67 A0 | A43 L67 L72 | A40 L68 L69 | L69 L68 A40 | L79 L74 A49 | A49 L74 L79 | A0 L81 A54 | A46 L75 L76 | L76 L75 A46 | L86 A50 A0 | A0 A50 L86 | A54 L81 A0 | A0 A50 L86 A55 L81 A54 | A0 L87 L88 A60 | L93 A56 A0 | A0 A56 L93 | A0 A58 L89 A57 L88 A61 L93 A56 | L89 A58 A0 | A0 A60 L88 L87 | A0 A56 L93 A61 L88 A60 | L100 L95 A67 | A67 L95 L100 | A63 L95 L96 | L96 L95 A63 | A66 L95 L94 | L94 L95 A66 | L107 L102 A73 | A73 L102 L107 | A72 L102 L101 | L101 L102 A72 | L114 L109 A79 | A79 L109 L114 | A75 L109 L110 | L110 L109 A75 | L121 L116 A85 | A85 L116 L121 | A84 L116 L115 | L115 L116 A84 | A81 L116 L117 | L117 L116 A81 | L128 A86 A0 | A0 A86 L128 | A86 L128 A91 L123 A90 L122 A89 A0 | L124 L123 A87 A0 | A0 A87 L123 L124 | A87 L123 A91 L128 A86 A0 | A0 A89 L122 | L135 A92 A0 | A0 A92 L135 | A93 L130 A97 L135 A92 A0 | A0 L130 A93 | L142 L137 A103 | A103 L137 L142 | A93 L130 A0 | A101 L136 L139 | L139 L136 A101 | A0 L144 L149 A109 | L149 L144 A109 | A107 L143 L146 | L146 L143 A107 | A113 L150 L153 | L153 L150 A113 | A0 A116 | L163 A116 A0 | A116 A0 L158 A120 L157 A119 L160 A118 | A0 A118 L160 | A0 A122 | L170 A122 A0 | L46 A21 A0 | A0 A21 L47 L46 | L165 L164 A126 A0 | A0 A126 L165 | A27 L54 L53 | L53 L54 A27 | A22 L47 L48 | L48 L47 A22 | A33 L61 L60 | L60 L61 A33 | A28 L54 L55 | L55 L54 A28 | A51 L81 L82 | L82 L81 A51 | A57 L88 L89 | L89 L88 A57 | A90 L123 L122 | L122 L123 A90 | A96 L130 L129 | L129 L130 A96 | A114 L150 L151 | L151 L150 A114 | A119 L157 L160 | L160 L157 A119 | A120 L157 L158 | L158 L157 A120 | A125 L164 L167 | L167 L164 A125 | A39 L68 L67 | L67 L68 A39 | A45 L75 L74 | L74 L75 A45 | A55 L86 L81 | A55 L81 L86 | A61 L93 L88 | A61 L88 L93 | L128 L123 A91 | A91 L123 L128 | L135 L130 A97 | A97 L130 L135 | A102 L136 L137 | L137 L136 A102 | A108 L143 L144 | L144 L143 A108 picked at (74.1105, -0.4081) picked at (74.1105, 0.4081) picked at (0.5059, 79.9894) picked at (0.5059, -79.9894)
extrude "Extrusion4" cut sketch "Sketch2" against normal blind 2 contours A7 L25 L0 | L0 L25 A7 | L25 A7 L0 | L0 A7 L25 | L37 L32 A13 | A13 L32 L37 | A13 L32 | L184 L179 A139 | A139 L179 L184 | L179 A139 | A19 L39 | L39 L44 A19 | A133 L177 L172 | L172 A133 | A19 L44 L39 | L172 L177 A133 | A25 L51 L46 | L46 A25 | A31 L58 L53 | L53 A31 | A121 L158 | L158 L163 A121 | A127 L165 | L165 L170 A127 | L51 A25 L46 | L58 A31 L53 | L65 L60 A37 | A37 L60 L65 | L60 A37 | A43 A0 L67 | L67 A0 A43 | A109 A0 L144 | L144 A0 A109 | L156 L151 A115 | A115 L151 L156 | A115 L151 | L158 A121 L163 | L165 A127 L170 | A0 L67 A43 | A43 L72 L67 A0 | A43 L67 L72 | L79 L74 A49 | A49 L74 L79 | L74 A49 | L100 L95 A67 | A67 L95 L100 | L107 L102 A73 | A73 L102 L107 | L114 L109 A79 | A79 L109 L114 | L121 L116 A85 | A85 L116 L121 | L142 L137 A103 | A103 L137 L142 | A103 L137 | A0 L144 L149 A109 | L149 L144 A109 | A0 A109 L144 | A73 L102 | L109 A79 | A67 L95 | L116 A85 | A55 L86 L81 | L81 A55 | A55 L81 L86 | A61 L93 L88 | L88 A61 | A61 L88 L93 | L128 L123 A91 | A91 L123 L128 | A91 L123 | L135 L130 A97 | A97 L130 L135 | A97 L130
extrude "Extrusion5" cut sketch "Sketch2" against normal through all contours L0 A2 A0 | L23 A2 A0 | A0 A2 L0 | A0 A2 L23 | A8 L37 A0 | A0 A8 | A134 A0 | A0 L184 A134 | L1 A8 A0 | L37 A8 L1 | A0 A134 L22 | L22 A134 L184 | A32 A0 L5 | L5 L65 A32 | A38 A0 L6 | L6 A0 A38 | A44 A0 L7 | L7 A0 A44 | A62 A0 L10 | L10 A0 A62 | A68 A0 L11 | L11 A0 A68 | A74 A0 L12 | L12 A0 A74 | A80 A0 L13 | L13 A0 A80 | A98 A0 L16 | L16 A0 A98 | A104 A0 L17 | L17 A0 A104 | A110 L156 L18 | L18 A0 A110 | A0 A32 | A0 A32 L65 | L72 A38 A0 | A0 A38 L72 | L79 A44 A0 | A0 A44 L79 | L100 A62 A0 | A0 A62 L100 | L107 A68 A0 | A0 A68 L107 | L114 A74 A0 | A0 A74 L114 | L121 A80 A0 | A0 A80 L121 | L142 A98 A0 | A0 A98 L142 | L149 A104 A0 | A0 A104 L149 | A0 A110 | L156 A110 A0 | A14 L44 A0 | A0 A14 | A128 A0 | A0 L177 A128 | A14 A0 L2 | L2 L44 A14 | A128 L177 L21 | L21 A0 A128 | A20 A0 L3 | L3 L51 A20 | A26 A0 L4 | L4 L58 A26 | A50 A0 L8 | L8 A0 A50 | A56 A0 L9 | L9 A0 A56 | A86 A0 L14 | L14 A0 A86 | A92 A0 L15 | L15 A0 A92 | A116 L163 L19 | L19 A0 A116 | A122 L170 L20 | L20 A0 A122 | A0 A20 | A0 A20 L51 | A0 A26 | A0 A26 L58 | L86 A50 A0 | A0 A50 L86 | L93 A56 A0 | A0 A56 L93 | L128 A86 A0 | A0 A86 L128 | L135 A92 A0 | A0 A92 L135 | A0 A116 | L163 A116 A0 | A0 A122 | L170 A122 A0
sketch "Sketch3" plane through (0, 0, 12) normal (0, 0, 1) x (1, 0, 0)
  circle A0 centre (0, 0) radius 107.5
  circle A1 centre (0, 107.5) radius 2.15
  circle A2 centre (-76.014, 76.014) radius 2.15
  circle A3 centre (-107.5, 0) radius 2.15
  circle A4 centre (-76.014, -76.014) radius 2.15
  circle A5 centre (0, -107.5) radius 2.15
  circle A6 centre (76.014, -76.014) radius 2.15
  circle A7 centre (107.5, 0) radius 2.15
  circle A8 centre (76.014, 76.014) radius 2.15
  dimension "d121" = 215
  dimension "d122" = 4.3
  dimension "d125" = 360
  constraints: 8 centre point, 1 coincident, 1 vertical alignment, 19 other
  measures "d122" diameter of A1
extrude "Extrusion6" cut sketch "Sketch3" against normal through all contours A0 A7 | A0 A7 | A8 A0 | A0 A8 | A6 A0 | A0 A6 | A1 A0 | A0 A1 | A5 A0 | A0 A5 | A2 A0 | A0 A2 | A4 A0 | A0 A4 | A3 A0 | A0 A3
sketch "Sketch4" plane through (0, 0, 14) normal (0, 0, 1) x (1, 0, 0)
  circle A0 centre (0, 0) radius 91
  line L0 (0, 0) -> (6.3478, 90.7783)
  line L1 (0, 168) -> (0, -168) projected
  circle A1 centre (6.3478, 90.7783) radius 2.1
  circle A2 centre (-67.0155, 61.5623) radius 2.1
  circle A3 centre (-89.9149, -14.0114) radius 2.1
  circle A4 centre (-45.1064, -79.0342) radius 2.1
  circle A5 centre (33.668, -84.5427) radius 2.1
  circle A6 centre (0, 0) radius 65
  line L2 (0, 0) -> (32.2189, 56.453)
  circle A7 centre (32.2189, 56.453) radius 2.1
  circle A8 centre (-24.0486, 60.3876) radius 2.1
  circle A9 centre (-62.207, 18.8491) radius 2.1
  circle A10 centre (-53.5223, -36.8832) radius 2.1
  circle A11 centre (-4.5342, -64.8417) radius 2.1
  circle A12 centre (87.0898, -26.3888) radius 2.1
  circle A13 centre (74.9312, 51.6364) radius 2.1
  circle A14 centre (47.8682, -43.9731) radius 2.1
  circle A15 centre (64.2249, 10.0081) radius 2.1
  dimension "d129" = 182
  dimension "d141" = 130
  dimension "d135" = 4
  dimension "d136" = 4.2
  dimension "d139" = 360
  dimension "d142" = 29.714
  dimension "d143" = 4.2
  dimension "d146" = 360
  constraints: 14 centre point, 4 coincident, 4 end point, 36 other
  measures "d135" angle of L1 L0
  measures "d136" diameter of A1
  measures "d142" angle of L1 L2
  measures "d143" diameter of A7
extrude "Extrusion7" cut sketch "Sketch4" against normal blind 8 contours A13 A0 | A0 A13 | A12 A0 | A0 A12 | A1 L0 A0 | A0 A1 | A5 A0 | A0 A5 | L0 A1 A0 | A7 A6 | A6 L2 A7 | A4 A0 | A0 A4 | A2 A0 | A0 A2 | L2 A6 A7 | A8 A6 | A6 A8 | A11 A6 | A6 A11 | A14 A6 | A6 A14 | A3 A0 | A0 A3 | A15 A6 | A6 A15 | A9 A6 | A6 A9 | A10 A6 | A6 A10
sketch "Sketch5" plane through (0, 0, 12) normal (0, 0, 1) x (1, 0, 0)
  line L0 (0, 168) -> (0, -168) projected
  line L1 (69.5236, 89.2106) -> (69.1253, 88.631)
  line L2 (71.3254, 84.4568) -> (66.4388, 77.6061)
  line L3 (9.2853, 110.1546) -> (7.8959, 101.8516)
  line L4 (13.9208, 112.2421) -> (13.7927, 111.5505)
  arc A0 (11.4618, 111.8141) -> (9.2853, 110.1546) centre (11.2579, 109.8245) ccw
  arc A1 (63.5351, 77.2224) -> (9.6749, 99.5309) centre (0, 0) ccw
  arc A2 (69.0767, 91.9424) -> (16.1685, 113.8577) centre (0, 0) ccw
  arc A3 (13.7927, 111.5505) -> (11.4618, 111.8141) centre (0, 0) ccw
  arc A4 (70.9598, 87.1692) -> (69.1253, 88.631) centre (0, 0) ccw
  arc A5 (16.1685, 113.8577) -> (13.9208, 112.2421) centre (15.8873, 111.8776) ccw
  arc A6 (7.8959, 101.8516) -> (9.6749, 99.5309) centre (9.8684, 101.5215) ccw
  arc A7 (63.5351, 77.2224) -> (66.4388, 77.6061) centre (64.8079, 78.7694) ccw
  arc A8 (71.3254, 84.4568) -> (70.9598, 87.1692) centre (69.6971, 85.6182) ccw
  arc A9 (69.5236, 89.2106) -> (69.0767, 91.9424) centre (67.8754, 90.3434) ccw
  line L5 (0, 0) -> (41.1385, 99.317)
  arc A10 (71.651, 84.2245) -> (71.2123, 87.4794) centre (69.6971, 85.6182) ccw
  line L6 (71.651, 84.2245) -> (66.7645, 77.3738)
  arc A11 (63.2809, 76.9135) -> (66.7645, 77.3738) centre (64.8079, 78.7694) ccw
  arc A12 (63.2809, 76.9135) -> (9.6362, 99.1328) centre (0, 0) ccw
  arc A13 (7.5013, 101.9176) -> (9.6362, 99.1328) centre (9.8684, 101.5215) ccw
  line L7 (7.5013, 101.9176) -> (8.8908, 110.2206)
  arc A14 (11.5026, 112.212) -> (8.8908, 110.2206) centre (11.2579, 109.8245) ccw
  arc A15 (13.4679, 111.9931) -> (11.5026, 112.212) centre (0, 0) ccw
  line L8 (13.4679, 111.9931) -> (13.5275, 112.3149)
  arc A16 (16.2248, 114.2537) -> (13.5275, 112.3149) centre (15.8873, 111.8776) ccw
  arc A17 (69.317, 92.2622) -> (16.2248, 114.2537) centre (0, 0) ccw
  arc A18 (69.8533, 88.9841) -> (69.317, 92.2622) centre (67.8754, 90.3434) ccw
  line L9 (69.8533, 88.9841) -> (69.6679, 88.7143)
  arc A19 (71.2123, 87.4794) -> (69.6679, 88.7143) centre (0, 0) ccw
  point P0 (0, 0)
  point P1 (70.9598, 87.1692)
  point P2 (71.2123, 87.4794)
  dimension "d151" = 22.5
  constraints: 1 other
extrude "Extrusion9" cut sketch "Sketch5" against normal through all contours L1 A4 A8 L2 A7 A1 A6 L3 A0 A3 L4 A5 A2 A9 | L6 A11 A12 A13 L7 A14 A15 L8 A16 A17 A18 L9 A19 A10
pattern_circular "Circular Pattern2" count 8 over 360 about axis through (0, 0, -10) along (0, 0, 1) of "Extrusion9"
sketch "Block2" plane through (0, 0, 0) normal (0, 0, 1) x (1, 0, 0)
  line L0 (83.1381, 5.88) -> (71.258, 5.88)
  line L1 (71.258, 5.88) -> (71.258, -6)
  line L2 (71.258, -6) -> (83.1381, -6)
  line L3 (83.1381, -6) -> (83.1381, 5.88)
  line L4 (83.1381, 5.88) -> (71.258, -6) construction
  line L5 (71.258, 5.88) -> (83.1381, -6) construction
  circle A0 centre (77.198, -0.06) radius 2
  circle A1 centre (72.671, -4.587) radius 2.1
  circle A2 centre (81.725, -4.587) radius 2.1
  circle A3 centre (81.725, 4.467) radius 2.1
  circle A4 centre (72.671, 4.467) radius 2.1
  circle A5 centre (70.898, -0.06) radius 0.75
  line L6 (70.898, -0.06) -> (77.198, -0.06)
  dimension "d13" = 11.88
  dimension "d15" = 4.2
  dimension "d21" = 360
  dimension "d22" = 142.521
  dimension "d23" = 0
  dimension "d24" = 45
  dimension "d25" = 90
  dimension "d26" = 135
  dimension "d27" = 180
  dimension "d28" = -45
  dimension "d29" = 90
  dimension "d30" = 135
  dimension "d31" = 180
  dimension "d32" = -45
  dimension "d33" = 90
  dimension "d34" = 135
  dimension "d35" = 0
  dimension "d36" = -45
  dimension "d37" = 90
  dimension "d38" = 45
  dimension "d39" = 140.97
  dimension "d40" = 360
  dimension "d41" = 0
  dimension "d42" = -32.727
  dimension "d12" = 11.88
  dimension "d14" = 4
  dimension "d16" = 1.413
  dimension "d17" = 360
  dimension "d18" = 1.5
  dimension "d19" = 6.3
  constraints: 6 end point, 2 centre point, 2 coincident, 2 midpoint, 1 horizontal, 1 point on line, 21 other
  measures "d12" distance of L5.end L4.end
  measures "d14" diameter of A0
  measures "d18" diameter of A5
  measures "d19" distance of L6.end L6.start
body "Solid1"
